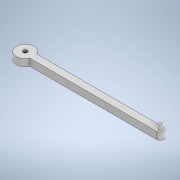
# Autodesk Inventor part: eslabon1
Saved by Autodesk Inventor 2021 (Build 250183000, 183)
## iProperties
Created: 2022-10-24
Part Number: eslabon1
Material: Generic
Document SubType Name: Modeling
Designer: felip
Density: 1 g/cm^3
Appearance: Default
Author: felip
Autodesk Inventor part; units mm, degrees
ref_plane "YZ Plane" through (0, 0, 0) normal (1, 0, 0) x (0, 1, 0)
ref_plane "XZ Plane" through (0, 0, 0) normal (0, 1, 0) x (-1, 0, 0)
ref_plane "XY Plane" through (0, 0, 0) normal (0, 0, 1) x (1, 0, 0)
sketch "Sketch1" plane through (0, 0, 0) normal (0, 1, 0) x (-1, 0, 0)
  arc A0 (0, 5) -> (0, -5) centre (0, 0) ccw
  arc A1 (-1.6, 1.2) -> (1.6, 1.2) centre (0, 0) ccw
  line L0 (-1.6, 1.2) -> (1.6, 1.2)
  line L1 (95, 124.2688) -> (95, -104.3981) construction
  circle A2 centre (190, 0) radius 11
  arc A3 (178.5436, -5) -> (178.5436, 5) centre (190, 0) ccw
  line L2 (0, -5) -> (178.5436, -5)
  line L3 (0, 5) -> (178.5436, 5)
  dimension "d2" = 10
  dimension "d3" = 4
  dimension "d4" = 1.2
  dimension "d5" = 95
  dimension "d8" = 22
  dimension "d9" = 25
  constraints: 8 end point, 6 point on circle, 4 centre point, 4 coincident, 2 horizontal, 1 parallel, 1 vertical
  measures "d2" diameter of A0
  measures "d3" diameter of A1
  measures "d4" distance from line of L0 point (0, 0)
  measures "d5" distance from line of point (0, 0) L1
  measures "d8" diameter of A2
  measures "d9" diameter of A3
extrude "Extrusion2" add sketch "Sketch1" along normal blind 10
sketch "Sketch2" plane through (0, 10, 0) normal (0, 1, 0) x (1, 0, 0)
  circle A0 centre (0, 0) radius 2.35
  dimension "d12" = 4.7
  constraints: 1 centre point, 1 coincident
  measures "d12" diameter of A0
extrude "Extrusion3" add sketch "Sketch2" along normal blind 7
sketch "Sketch3" plane through (0, 10, 0) normal (0, 1, 0) x (1, 0, 0)
  circle A0 centre (-190, 0) radius 11 construction
  line L0 (-179, 0) -> (-201, 0) construction
  circle A1 centre (-190, 0) radius 11
  circle A2 centre (-190, 0) radius 3
  point P0 (0, 0)
  dimension "d15" = 22
  dimension "d16" = 22
  dimension "d17" = 6
  constraints: 3 coincident, 2 centre point, 2 end point, 2 point on circle, 1 horizontal
  measures "d15" distance of L0.start L0.end
  measures "d16" diameter of A1
  measures "d17" diameter of A2
extrude "Extrusion4" add sketch "Sketch3" against normal blind 3
equation "\"d16\" = d15"
body "Solid2"
